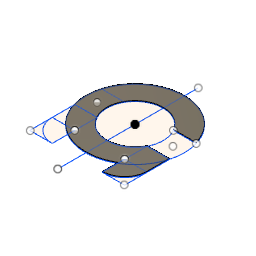
PolytechLogo (Autodesk Fusion 360 design; units mm, degrees)
Autodesk Fusion 360 part; units mm, degrees
note: some values were not read from the file. Set by a fixed rule: which sketch regions a step uses.
sketch "Sketch1" plane through (0, 0, 0) normal (0, 1, 0) x (1, 0, 0)
  circle A0 centre (0, 0) radius 35
  circle A1 centre (0, 0) radius 20
  line L0 (-17.3205, 10) -> (-33.541, 10)
  line L1 (-17.7813, -9.1557) -> (-33.7813, -9.1557)
  line L2 (-17.7813, -9.1557) -> (-33.7813, -9.1557)
  line L3 (-33.7813, -9.1557) -> (-33.7813, -41.1557)
  line L4 (-33.7813, -41.1557) -> (-17.7813, -41.1557)
  line L5 (-17.7813, -41.1557) -> (-17.7813, -9.1557)
  line L6 (-17.7813, -41.1557) -> (-33.4653, -41.1557)
  line L7 (-17.7813, -25.1557) -> (-17.7813, -41.1557)
  line L8 (-17.7813, -41.1557) -> (-33.7813, -41.1557)
  line L9 (-33.7813, -41.1557) -> (-33.7813, -25.1557)
  line L10 (-33.7813, -25.1557) -> (-17.7813, -25.1557)
  line L11 (-17.7813, -25.1557) -> (-17.7813, -41.1557)
  arc A2 (-33.7813, -25.1557) -> (-17.7813, -41.1557) centre (-17.7813, -25.1557) ccw
  line L12 (0, 45) -> (0, -55)
  line L13 (17.7813, -25.1557) -> (17.7813, -41.1557)
  line L14 (17.7813, -25.1557) -> (17.7813, -41.1557)
  arc A3 (17.7813, -41.1557) -> (33.7813, -25.1557) centre (17.7813, -25.1557) ccw
  line L15 (17.3205, 10) -> (33.541, 10)
  line L16 (17.7813, -9.1557) -> (33.7813, -9.1557)
  line L17 (33.7813, -41.1557) -> (33.7813, -25.1557)
  line L18 (33.7813, -9.1557) -> (33.7813, -41.1557)
  line L19 (17.7813, -41.1557) -> (33.4653, -41.1557)
  line L20 (17.7813, -9.1557) -> (33.7813, -9.1557)
  line L21 (17.7813, -41.1557) -> (33.7813, -41.1557)
  line L22 (17.7813, -41.1557) -> (17.7813, -9.1557)
  circle A4 centre (0, 0) radius 20
  circle A5 centre (0, 0) radius 35
  line L23 (33.7813, -25.1557) -> (17.7813, -25.1557)
  line L24 (33.7813, -41.1557) -> (17.7813, -41.1557)
  point P0 (-27, 0)
  point P1 (0, -55)
  point P2 (27, 0)
  dimension "d1" = 70
  dimension "d3" = 32
  dimension "d4" = 16
  constraint coincident A0.centre A1.centre
  constraint concentric A0 A1
  constraint coincident A0 L0.end
  constraint horizontal L0
  constraint coincident A0 L1.end
  constraint parallel L0 L1
  constraint coincident A1 L0.start
  constraint coincident A1 L1.start
  constraint perpendicular L2 L3
  constraint parallel L2 L4
  constraint parallel L3 L5
  constraint parallel L1 L2
  constraint horizontal L6
  constraint vertical L7
  constraint horizontal L8
  constraint vertical L9
  constraint horizontal L10
  constraint vertical L11
  constraint midpoint L3 L9.end
  constraint vertical L12
  constraint symmetric A0.centre L12 A1.centre
  constraint symmetric A0 L12 A5
  constraint symmetric A1 L12 A4
  constraint symmetric P0 L12 P2
  constraint symmetric L0.start L12 L15.start
  constraint symmetric L0.end L12 L15.end
  constraint symmetric L1.start L12 L16.start
  constraint symmetric L1.end L12 L16.end
  constraint symmetric L3.end L12 L17.start
  constraint symmetric L4.end L12 L13.end
  constraint symmetric L6.end L12 L19.end
  constraint symmetric L7.start L12 L13.start
  constraint symmetric L9.end L12 A3.end
  constraint symmetric A2 L12 A3
  constraint symmetric P1 L12 L12.end
  measures "d1" diameter of A0
  measures "d3" distance of L1.end L3.end
  measures "d4" distance of L3.end L4.end
extrude "Extrude2" add sketch "Sketch1" along normal blind 0.6 contours A0 A1 L12 L15 A4 A5 | A0 L18 A5 L23 | A0 L16 L20 L22 A5 L23 | A0 A1 L0 L12 A4 A5 | A0 L13 L14 A3 L22 A5 L23 | A0 L13 L14 L22 A5 L23 | A0 A1 L12 L13 L14 L22 A4 A5 | A0 A1 L0 L1 L2 A4 A5 | A0 A1 L5 L7 L11 L12 A4 A5 | A0 L1 L2 L5 L10 A5 | A0 L5 L7 L10 L11 A5 makes body 1
extrude "Extrude1" add sketch "Sketch1" along normal blind 0.6 separate body contours A0 A1 L15 L16 L20 A4 A5 | A0 A1 L12 L15 A4 A5 | A0 L16 L20 L22 A5 L23 | A0 A1 L0 L12 A4 A5 | A0 L13 L14 L22 A5 L23 | A0 A1 L12 L13 L14 L22 A4 A5 | A0 A1 L5 L7 L11 L12 A4 A5 | A0 L1 L2 L5 L10 A5 | A0 L3 L10 A5 | A0 L5 L7 L10 L11 A5 | A0 L5 L7 L10 L11 A2 A5 makes body 2
sketch "Sketch2" plane through (0, 0, 0) normal (0, 1, 0) x (1, 0, 0)
hidden bodies 2
